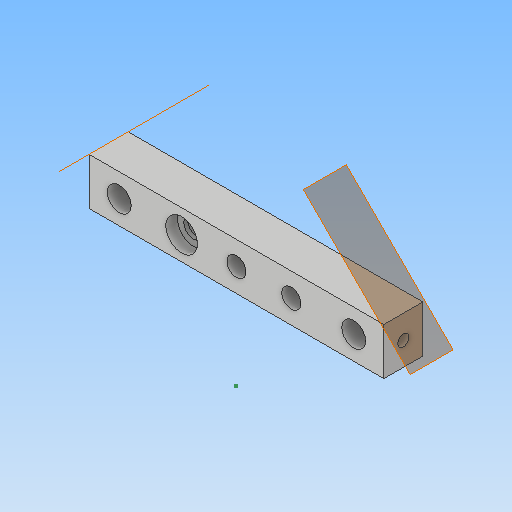
# Autodesk Inventor part: cellSTORM_inverted_sampleholder_bar
Saved by Autodesk Inventor 2019.4 (Build 234330000, 330)
## iProperties
Created: 2020-11-05
Part Number: cellSTORM_inverted_sampleholder_bar
Material: Generic
Document SubType Name: Modeling
Designer: diederichbenedict
Density: 1 g/cm^3
Appearance: Default
Author: diederichbenedict
Autodesk Inventor part; units mm, degrees
ref_plane "YZ Plane" through (0, 0, 0) normal (1, 0, 0) x (0, 1, 0)
ref_plane "XZ Plane" through (0, 0, 0) normal (0, 1, 0) x (-1, 0, 0)
ref_plane "XY Plane" through (0, 0, 0) normal (0, 0, 1) x (1, 0, 0)
sketch "Sketch1" plane through (0, 0, 0) normal (0, 0, 1) x (1, 0, 0)
  circle A0 centre (30, 26.4525) radius 3 projected
  circle A1 centre (-30, 26.4525) radius 3 projected
  line L0 (-12, 6.73) -> (12, 6.73) projected
  line L1 (12, 6.73) -> (12, 13) projected
  line L2 (12, 13) -> (-12, 13) projected
  line L3 (-12, 13) -> (-12, 6.73) projected
  line L4 (0, 33.0213) -> (0, 0)
  circle A2 centre (30, 26.4525) radius 3.05
  circle A3 centre (-30, 26.4525) radius 3.05
  line L5 (37.7199, 32.4525) -> (0, 32.4525)
  line L6 (0, 32.4525) -> (0, 20.4525)
  line L7 (0, 20.4525) -> (37.7199, 20.4525)
  line L8 (37.7199, 20.4525) -> (37.7199, 32.4525)
  circle A4 centre (30, 26.4525) radius 6 construction
  dimension "d0" = 6.1
  dimension "d1" = 6.1
  dimension "d12" = 3
  constraints: 10 end point, 3 centre point, 2 coincident, 2 parallel, 2 tangent, 1 horizontal, 1 perpendicular, 1 point on line, 1 vertical
  measures "d0" diameter of A2
  measures "d1" diameter of A3
  measures "d12" radial gap between concentric circles of A0 A4
extrude "Extrusion1" add sketch "Sketch1" against normal blind 10 contours L5 L8 L7 L4
sketch "Sketch2" plane through (0, 0, 0) normal (0, 0, 1) x (1, 0, 0)
  circle A0 centre (30, 26.4525) radius 3.05 projected
  line L0 (0, 20.4525) -> (0, 32.4525) projected
  circle A1 centre (0, 26.4525) radius 2.45
  circle A2 centre (14.0354, 26.4525) radius 2.45
  dimension "d13" = 4.9
  dimension "d14" = 4.9
  constraints: 2 centre point, 1 midpoint
  measures "d13" diameter of A1
  measures "d14" diameter of A2
extrude "Extrusion2" cut sketch "Sketch2" against normal blind 4 contours A1 L0 | L0 A1 | A2
sketch "Sketch3" plane through (37.7199, 20.4525, 0) normal (1, 0, 0) x (0, 0, -1)
  line L0 (0, 0) -> (0, 12) projected
  line L1 (0, 0) -> (10, 0) projected
  line L2 (10, 12) -> (10, 0) projected
  line L3 (0, 12) -> (10, 12) projected
  circle A0 centre (5, 6) radius 1.45
  point P0 (0, -20.4525)
  dimension "d15" = 2.9
  constraints: 1 centre point
  measures "d15" diameter of A0
extrude "Extrusion3" cut sketch "Sketch3" against normal up to surface contours A0 round surface about axis through (30, 26.4525, 0) along (0, 0, -1) radius 3.05 far side no
ref_plane "Work Plane1" through (37.7199, 32.4525, 0) normal (0.7071068, 0.7071068, 0) x (0, 0, 1)
mirror "Mirror2" about plane through (0, 20.4525, 0) normal (-1, 0, 0) of "Extrusion1", "Extrusion2", "Extrusion3"
sketch "Sketch5" plane through (0, 0, 0) normal (0, 0, 1) x (1, 0, 0)
  point P0 (0, 0)
sketch "Sketch6" plane through (0, 0, 0) normal (0, 0, 1) x (1, 0, 0)
  circle A0 centre (-14.0354, 26.4525) radius 2.45 projected
  circle A1 centre (-14.0354, 26.4525) radius 4.05
  point P0 (0, 0)
  dimension "d31" = 8.1
  constraints: 1 centre point, 1 coincident
  measures "d31" diameter of A1
extrude "Extrusion5" cut sketch "Sketch6" against normal blind 3 contours A0 | A1
ref_plane "Work Plane2" through (-37.7199, 32.4525, 0) normal (0.7071068, -0.7071068, 0) x (0, 0, 1)
body "Solid1"
